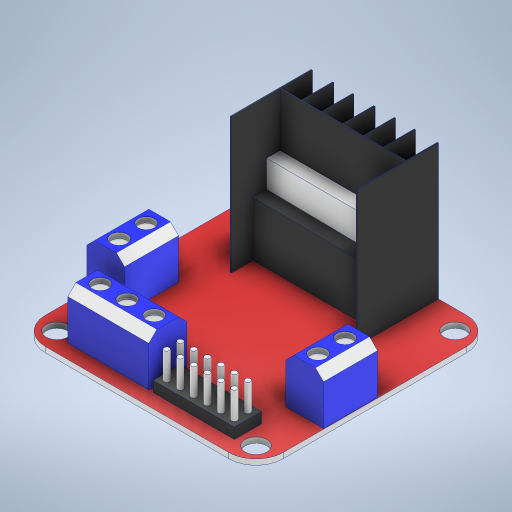
# Autodesk Inventor part: Ponte_H
Saved by Autodesk Inventor 2023 (Build 270158000, 158)
## iProperties
Created: 2023-03-21
Part Number: Ponte_H
Material: Alumínio 6061
Document SubType Name: Sheet Metal
Designer: Antonio Ribeiro
Density: 2.7 g/cm^3
Sheet Metal Rule: Default_mm
Appearance: Alumínio - Plano
Author: Antonio Ribeiro
Autodesk Inventor part; units mm, degrees
ref_plane "YZ Plane" through (0, 0, 0) normal (1, 0, 0) x (0, 1, 0)
ref_plane "XZ Plane" through (0, 0, 0) normal (0, 1, 0) x (-1, 0, 0)
ref_plane "XY Plane" through (0, 0, 0) normal (0, 0, 1) x (1, 0, 0)
sketch "Esboço6" plane through (0, 0, 0) normal (0, 1, 0) x (-1, 0, 0)
  line L0 (0, -22) -> (-17, -22)
  line L1 (-22, -17) -> (-22, 17)
  line L2 (-17, 22) -> (17, 22)
  line L3 (22, 17) -> (22, -15.5)
  line L4 (15.5, -22) -> (0, -22)
  arc A0 (-22, -17) -> (-17, -22) centre (-17, -17) ccw
  arc A1 (-17, 22) -> (-22, 17) centre (-17, 17) ccw
  arc A2 (22, 17) -> (17, 22) centre (17, 17) ccw
  line L5 (15.5, -22) -> (17, -22)
  line L6 (22, -15.5) -> (22, -17)
  arc A3 (17, -22) -> (22, -17) centre (17, -17) ccw
  circle A4 centre (18.4142, -18.4142) radius 2
  circle A5 centre (18.4142, 18.4142) radius 2
  circle A6 centre (-18.4142, 18.4142) radius 2
  circle A7 centre (-18.4142, -18.4142) radius 2
  point P0 (0, 0)
  point P1 (-22, -22)
  point P2 (-22, 22)
  point P3 (22, 22)
  point P4 (22, -22)
  dimension "d23" = 22
  dimension "d24" = 22
  dimension "d25" = 44
  dimension "d26" = 44
  dimension "d28" = 5
  dimension "d29" = 5
  dimension "d31" = 4
  dimension "d35" = 4
  dimension "d36" = 4
  dimension "d37" = 4
  constraints: 14 end point, 11 point on line, 8 centre point, 8 point on circle, 8 tangent, 5 perpendicular, 2 equal radius, 1 horizontal
  measures "d23" distance of point (0, 0) L0.start
  measures "d24" distance of L0.start point (-22, -22)
  measures "d25" distance of point (-22, -22) point (-22, 22)
  measures "d26" distance of point (-22, 22) point (22, 22)
  measures "d28" radius of A0
  measures "d29" radius of A3
  measures "d31" diameter of A4
  measures "d35" diameter of A5
  measures "d36" diameter of A6
  measures "d37" diameter of A7
extrude "Extrusão4" add sketch "Esboço6" along normal blind 1
sketch "Esboço7" plane through (0, 1, 0) normal (0, 1, 0) x (1, 0, 0)
  circle A0 centre (-18.4142, -18.4142) radius 2 projected
  line L0 (-18.4142, -18.4142) -> (-16.4142, -18.4142)
  line L1 (-16.4142, -18.4142) -> (-16.4142, -19.4142)
  line L2 (-16.4142, -19.4142) -> (-15.4142, -19.4142)
  line L3 (-15.4142, -19.4142) -> (-0.4142, -19.4142)
  line L4 (-0.4142, -19.4142) -> (-0.4142, -12.4142)
  line L5 (-15.4142, -19.4142) -> (-15.4142, -12.4142)
  line L6 (-15.4142, -12.4142) -> (-0.4142, -12.4142)
  point P0 (0, 0)
  dimension "d40" = 1
  dimension "d41" = 1
  dimension "d42" = 15
  dimension "d43" = 7
  constraints: 14 end point, 4 perpendicular, 1 horizontal, 1 horizontal alignment, 1 point on line, 1 vertical, 1 other
  measures "d40" distance of L0.end L1.end
  measures "d41" distance of L1.end L2.end
  measures "d42" distance of L2.end L3.end
  measures "d43" distance of L3.end L4.end
extrude "Extrusão5" add sketch "Esboço7" along normal blind 9 contours L5 L6 L4 L3
chamfer "Chanfro1" distance 1.5 angle 45 2 edges at (-7.9142, 10, 19.4142) (-7.9142, 10, 12.4142)
sketch "Esboço8" plane through (0, 10, 0) normal (0, 1, 0) x (1, 0, 0)
  line L0 (-0.4142, -17.9142) -> (-0.4142, -13.9142) projected
  line L1 (-0.4142, -15.9142) -> (-15.4142, -15.9142)
  line L2 (-15.4142, -13.9142) -> (-15.4142, -17.9142) projected
  line L3 (-0.4142, -15.9142) -> (-5.4142, -15.9142)
  line L4 (-5.4142, -15.9142) -> (-10.4142, -15.9142)
  line L5 (-10.4142, -15.9142) -> (-15.4142, -15.9142)
  circle A0 centre (-2.9142, -15.9142) radius 1.5
  circle A1 centre (-7.9142, -15.9142) radius 1.5
  circle A2 centre (-12.9142, -15.9142) radius 1.5
  point P0 (0, 0)
  dimension "d49" = 5
  dimension "d50" = 5
  dimension "d51" = 3
  dimension "d52" = 3
  dimension "d53" = 3
  constraints: 8 end point, 5 midpoint, 3 centre point, 2 point on line, 1 collinear
  measures "d49" distance of L1.start L3.end
  measures "d50" distance of L3.end L4.end
  measures "d51" diameter of A0
  measures "d52" diameter of A1
  measures "d53" diameter of A2
extrude "Extrusão6" cut sketch "Esboço8" against normal blind 1
sketch "Esboço9" plane through (0, 1, 0) normal (0, 1, 0) x (1, 0, 0)
  circle A0 centre (18.4142, -18.4142) radius 2 projected
  line L0 (18.4142, -18.4142) -> (16.4142, -18.4142)
  line L1 (16.4142, -18.4142) -> (16.4142, -19.4142)
  line L2 (16.4142, -19.4142) -> (15.4142, -19.4142)
  line L3 (15.4142, -19.4142) -> (0.4142, -19.4142)
  line L4 (0.4142, -19.4142) -> (0.4142, -14.4142)
  line L5 (0.4142, -14.4142) -> (15.4142, -14.4142)
  line L6 (15.4142, -14.4142) -> (15.4142, -19.4142)
  point P0 (0, 0)
  dimension "d56" = 1
  dimension "d57" = 1
  dimension "d58" = 15
  dimension "d59" = 5
  constraints: 14 end point, 4 perpendicular, 1 horizontal, 1 horizontal alignment, 1 point on line, 1 vertical, 1 other
  measures "d56" distance of L0.end L1.end
  measures "d57" distance of L1.end L2.end
  measures "d58" distance of L2.end L3.end
  measures "d59" distance of L3.end L4.end
extrude "Extrusão7" add sketch "Esboço9" along normal blind 7 contours L3 L4 L5 L6
sketch "Esboço11" plane through (0, 8, 0) normal (0, 1, 0) x (1, 0, 0)
  line L0 (0.4142, -19.4142) -> (0.4142, -14.4142) projected
  line L1 (0.4142, -19.4142) -> (0.4142, -14.4142)
  line L2 (0.4142, -14.4142) -> (0.4142, -16.9142)
  line L3 (0.4142, -16.9142) -> (15.4142, -16.9142)
  line L4 (15.4142, -19.4142) -> (15.4142, -14.4142) projected
  line L5 (0.4142, -19.4142) -> (0.4142, -16.9142)
  circle A0 centre (1.6642, -18.1642) radius 0.5
  circle A1 centre (4.1642, -18.1642) radius 0.5
  circle A2 centre (6.6642, -18.1642) radius 0.5
  circle A3 centre (9.1642, -18.1642) radius 0.5
  circle A4 centre (11.6642, -18.1642) radius 0.5
  circle A5 centre (14.1642, -18.1642) radius 0.5
  circle A6 centre (1.6642, -15.6642) radius 0.5
  circle A7 centre (4.1642, -15.6642) radius 0.5
  circle A8 centre (6.6642, -15.6642) radius 0.5
  circle A9 centre (9.1642, -15.6642) radius 0.5
  circle A10 centre (11.6642, -15.6642) radius 0.5
  circle A11 centre (14.1642, -15.6642) radius 0.5
  line L6 (15.4142, -14.4142) -> (0.4142, -14.4142) projected
  line L7 (0.4142, -14.4142) -> (15.4142, -14.4142)
  line L8 (15.4142, -14.4142) -> (15.4142, -16.9142)
  line L9 (15.4142, -19.4142) -> (15.4142, -16.9142)
  line L10 (0.4142, -14.4142) -> (0.4142, -19.4142) projected
  line L11 (0.4142, -19.4142) -> (15.4142, -19.4142) projected
  line L12 (0.4142, -19.4142) -> (15.4142, -19.4142)
  point P0 (0, 0)
  dimension "d68" = 1
  dimension "d69" = 1
  dimension "d70" = 1
  dimension "d71" = 1
  dimension "d72" = 1
  dimension "d73" = 1
  constraints: 16 end point, 12 centre point, 6 symmetric about line, 5 collinear, 2 midpoint, 1 perpendicular, 6 other
  measures "d68" diameter of A0
  measures "d69" diameter of A1
  measures "d70" diameter of A2
  measures "d71" diameter of A3
  measures "d72" diameter of A4
  measures "d73" diameter of A5
extrude "Extrusão8" cut sketch "Esboço11" against normal blind 5
sketch "Esboço12" plane through (0, 1, 0) normal (0, 1, 0) x (1, 0, 0)
  circle A0 centre (-18.4142, -18.4142) radius 2 projected
  line L0 (-18.4142, -9.4142) -> (-14.9142, -9.4142)
  line L1 (-14.9142, -9.4142) -> (-14.9142, 0.5858)
  line L2 (-14.9142, 0.5858) -> (-18.4142, 0.5858)
  line L3 (-22, 17) -> (-22, -17) projected
  line L4 (-18.4142, 0.5858) -> (-21.9142, 0.5858)
  line L5 (-21.9142, 0.5858) -> (-21.9142, -9.4142)
  line L6 (-21.9142, -9.4142) -> (-18.4142, -9.4142)
  point P0 (0, 0)
  dimension "d77" = 10
  dimension "d78" = 3.5
  dimension "d79" = 3.5
  constraints: 12 end point, 3 perpendicular, 2 point on line, 1 collinear, 1 horizontal
  measures "d77" distance of L2.end L0.start
  measures "d78" distance of L0.start L0.end
  measures "d79" distance of L2.end L4.end
extrude "Extrusão9" add sketch "Esboço12" along normal blind 9 contours L6 L5 L4 L2 L1 L0
sketch "Esboço13" plane through (0, 10, 0) normal (0, 1, 0) x (1, 0, 0)
  line L0 (-14.9142, 0.5858) -> (-21.9142, 0.5858) projected
  line L1 (-18.4142, 0.5858) -> (-18.4142, -1.9142)
  line L2 (-18.4142, -1.9142) -> (-18.4142, -4.4142)
  line L3 (-18.4142, -4.4142) -> (-18.4142, -6.9142)
  circle A0 centre (-18.4142, -1.9142) radius 1.5
  circle A1 centre (-18.4142, -6.9142) radius 1.5
  point P0 (0, 0)
  point P1 (-16.9142, 0.5858)
  point P2 (-19.9142, 0.5858)
  dimension "d83" = 2.5
  dimension "d84" = 2.5
  dimension "d85" = 2.5
  dimension "d86" = 3
  dimension "d87" = 3
  constraints: 6 end point, 2 centre point, 2 coincident, 2 point on line, 1 midpoint, 1 vertical
  measures "d83" distance of L1.start L1.end
  measures "d84" distance of L1.end L2.end
  measures "d85" distance of L2.end L3.end
  measures "d86" diameter of A0
  measures "d87" diameter of A1
extrude "Extrusão10" cut sketch "Esboço13" against normal blind 1
chamfer "Chanfro2" distance 1.5 angle 45 2 edges at (-14.9142, 10, 4.4142) (-21.9142, 10, 4.4142)
sketch "Esboço14" plane through (0, 1, 0) normal (0, 1, 0) x (1, 0, 0)
  line L0 (-14.9142, 0.5858) -> (-14.9142, -9.4142) projected
  line L1 (-14.9142, -9.4142) -> (22, -9.4142)
  line L2 (22, -17) -> (22, 17) projected
  line L3 (-14.9142, 0.588) -> (22, 0.588)
  circle A0 centre (18.4142, -18.4142) radius 2 projected
  line L4 (18.4142, -9.4142) -> (21.9142, -9.4142)
  line L5 (21.9142, -9.4142) -> (21.9142, 0.588)
  line L6 (18.4142, -9.4142) -> (14.9142, -9.4142)
  line L7 (14.9142, -9.4142) -> (14.9142, 0.588)
  line L8 (21.9142, 0.588) -> (14.9142, 0.588)
  point P0 (0, 0)
  dimension "d93" = 3.5
  dimension "d94" = 3.5
  constraints: 14 end point, 6 point on line, 2 horizontal, 2 perpendicular, 1 collinear
  measures "d93" distance of L4.start L4.end
  measures "d94" distance of L4.start L6.end
extrude "Extrusão11" add sketch "Esboço14" along normal blind 9 contours L7 L3 L5 L1
chamfer "Chanfro3" distance 1.5 angle 45 2 edges at (21.9142, 10, 4.4131) (14.9142, 10, 4.4131)
sketch "Esboço16" plane through (0, 10, 0) normal (0, 1, 0) x (1, 0, 0)
  circle A0 centre (-18.4142, -1.9142) radius 1.5 projected
  line L0 (20.4142, 0.588) -> (20.4142, -9.4142) projected
  circle A1 centre (-18.4142, -6.9142) radius 1.5 projected
  circle A2 centre (18.4142, -6.9142) radius 1.5
  circle A3 centre (18.4142, -1.9142) radius 1.5
  point P0 (0, 0)
  dimension "d101" = 3
  dimension "d102" = 3
  constraints: 2 centre point
  measures "d101" diameter of A2
  measures "d102" diameter of A3
extrude "Extrusão12" cut sketch "Esboço16" against normal blind 1 contours A2 | A3
sketch "Esboço17" plane through (0, 1, 0) normal (0, 1, 0) x (1, 0, 0)
  circle A0 centre (-18.4142, 18.4142) radius 2 projected
  arc A1 (-17, 22) -> (-22, 17) centre (-17, 17) ccw projected
  circle A2 centre (18.4142, 18.4142) radius 2 projected
  arc A3 (22, 17) -> (17, 22) centre (17, 17) ccw projected
  line L0 (-11.7958, 18.4142) -> (-11.7958, 22)
  line L1 (17, 22) -> (-17, 22) projected
  line L2 (11.7958, 18.4142) -> (11.7958, 22)
  line L3 (-11.7958, 22) -> (-11.7958, 7)
  line L4 (11.7958, 7) -> (11.7958, 22)
  line L5 (-11.7958, 22) -> (11.7958, 22)
  line L6 (-10.7958, 16) -> (10.7958, 16)
  line L7 (-11.2958, 16) -> (10.7958, 16)
  line L8 (10.7958, 16) -> (11.2958, 16)
  line L9 (-11.7958, 7) -> (-11.5458, 7)
  line L10 (-11.5458, 7) -> (-11.5458, 16)
  line L11 (-11.5458, 16) -> (-11.2958, 16)
  line L12 (11.7958, 7) -> (11.5458, 7)
  line L13 (11.5458, 7) -> (11.5458, 16)
  line L14 (11.5458, 16) -> (11.2958, 16)
  line L15 (-11.5458, 16.25) -> (-11.5458, 22)
  line L16 (-11.7958, 22) -> (-11.5458, 22)
  line L17 (11.5458, 16.25) -> (11.5458, 22)
  line L18 (7.2792, 16.25) -> (7.2792, 22)
  line L19 (7.2792, 22) -> (7.5292, 22)
  line L20 (7.5292, 22) -> (7.4542, 16.25)
  line L21 (3.8292, 16.25) -> (3.8292, 22)
  line L22 (3.8292, 22) -> (3.5792, 22)
  line L23 (3.5792, 22) -> (3.5792, 16.25)
  line L24 (0.0292, 16.25) -> (0.0292, 22)
  line L25 (0.0292, 22) -> (-0.2208, 22)
  line L26 (-0.2208, 22) -> (-0.2208, 16.25)
  line L27 (-4.1208, 16.25) -> (-4.1208, 22)
  line L28 (-4.1208, 22) -> (-3.8708, 22)
  line L29 (-3.8708, 22) -> (-3.8708, 16.25)
  line L30 (-7.5708, 16.25) -> (-7.5708, 22)
  line L31 (-7.5708, 22) -> (-7.8208, 22)
  line L32 (-7.8208, 22) -> (-7.8208, 16.25)
  line L33 (11.5458, 16.25) -> (7.4542, 16.25)
  line L34 (7.2792, 16.25) -> (3.8292, 16.25)
  line L35 (3.5792, 16.25) -> (0.0292, 16.25)
  line L36 (-0.2208, 16.25) -> (-3.8708, 16.25)
  line L37 (-4.1208, 16.25) -> (-7.5708, 16.25)
  line L38 (-7.8208, 16.25) -> (-11.5458, 16.25)
  point P0 (0, 0)
  dimension "d107" = 15
  dimension "d122" = 0.25
  dimension "d124" = 0.25
  dimension "d126" = 0.25
  dimension "d128" = 0.25
  dimension "d130" = 0.25
  constraints: 74 end point, 7 perpendicular, 6 parallel, 4 vertical, 3 collinear, 3 point on line, 1 horizontal, 15 other
  measures "d107" distance of L0.end L3.end
  measures "d122" distance of L18.end L19.end
  measures "d124" distance of L21.end L22.end
  measures "d126" distance of L24.end L25.end
  measures "d128" distance of L27.end L28.end
  measures "d130" distance of L30.end L31.end
extrude "Extrusão13" add sketch "Esboço17" along normal blind 25 contours L0 L1 L15 L38 L32 L30 L37 L27 L29 L36 L26 L24 L35 L23 L21 L34 L18 L20 L33 L17 L2 L4 L12 L13 L14 L8 L6 L7 L11 L10 L9 L3
sketch "Esboço20" plane through (-11.5458, 1, -16) normal (0, 0, 1) x (1, 0, 0)
  line L0 (23.0917, 0) -> (0, 0) projected
  line L1 (11.575, 10) -> (0, 10.1493)
  line L2 (0, 0) -> (0, 25) projected
  line L3 (11.575, 10) -> (23.0917, 9.8514)
  line L4 (23.0917, 0) -> (23.0917, 25) projected
  line L5 (23.0917, 9.8514) -> (23.0917, 0)
  line L6 (23.0917, 0) -> (11.575, 0)
  line L7 (0, 10.1493) -> (0, 0)
  line L8 (11.575, 0) -> (15.125, 0) projected
  line L9 (0, 0) -> (11.575, 0)
  line L10 (11.575, 0) -> (0, 0)
  point P0 (11.5458, -1)
  constraints: 14 end point, 3 collinear, 3 point on line
extrude "Extrusão14" add sketch "Esboço20" along normal blind 5
sketch "Esboço21" plane through (-11.5458, 26, -16) normal (0, 0, 1) x (1, 0, 0)
  line L0 (0, -14.8507) -> (0, -9.8507)
  line L1 (0, -14.8507) -> (0, 0) projected
  line L2 (0, -9.8507) -> (23.0917, -9.8507)
  line L3 (23.0917, -15.1486) -> (23.0917, 0) projected
  line L4 (23.0917, -9.8507) -> (23.0917, -15.1486)
  line L5 (23.0917, -15.1486) -> (0.4734, -14.8507)
  line L6 (0, -14.8507) -> (23.0917, -15.1486) projected
  line L7 (23.0917, -15.1486) -> (0, -14.8507)
  point P0 (11.5458, -26)
  dimension "d136" = 5
  constraints: 10 end point, 2 point on line, 1 collinear, 1 perpendicular
  measures "d136" distance of L0.start L0.end
extrude "Extrusão15" add sketch "Esboço21" along normal blind 2.5
equation "\"Raio_vergadura\" = Espessura"
equation "\"Largura_alívio_de_vergadura\" = Espessura"
equation "\"Profundidade_alívio_de_vergadura\" = 0.5 * Espessura"
equation "\"Tamanho_alívio_de_dobra\" = 4 * Espessura"
equation "\"Remanescente_mínimo\" = 2 * Espessura"
equation "\"Raiodetransição\" = Raio_vergadura"
equation "\"Tamanho_de_raio_de_Jacobi\" = Raio_vergadura"
equation "\"TamanhoFolga\" = Espessura"
equation "\"Espessura\" = 0.5"
